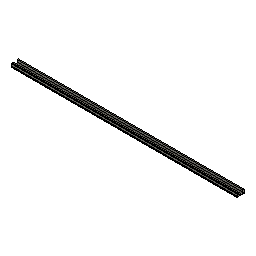
Extrusion Cover v6 200mm (Autodesk Fusion 360 design; units mm, degrees)
Autodesk Fusion 360 part; units mm, degrees
sketch "Sketch1" plane through (0, 0, 0) normal (1, 0, 0) x (0, 1, 0) in component "Cover"
sketch "Sketch2" plane through (0, 0, 0) normal (1, 0, 0) x (0, 1, 0) in component "Cover"
  line L0 (-3.5, -0.405) -> (3.5, -0.405)
  line L1 (-3.5, -0.405) -> (-3.5, -0.005)
  line L2 (3.5, -0.405) -> (3.5, -0.005)
  line L3 (-3, -0.005) -> (-3, 1.895)
  line L4 (3, -0.005) -> (3, 1.895)
  line L5 (-1.8, -0.005) -> (-1.8, 1.895)
  line L6 (1.8, -0.005) -> (1.8, 1.895)
  line L7 (-1.8, 1.895) -> (-1.8, 2.795)
  line L8 (1.8, 1.895) -> (1.8, 2.795)
  line L9 (-1.8, 2.795) -> (-3.2, 2.795)
  line L10 (1.8, 2.795) -> (3.2, 2.795)
  line L11 (-3, 1.895) -> (-3.2, 1.895)
  line L12 (3, 1.895) -> (3.2, 1.895)
  line L13 (-3.2, 2.795) -> (-3.2, 1.895)
  line L14 (3.2, 2.795) -> (3.2, 1.895)
  line L15 (-3.5, -0.005) -> (-3, -0.005)
  line L16 (-1.8, -0.005) -> (1.8, -0.005)
  line L17 (3, -0.005) -> (3.5, -0.005)
  dimension "d6" = 7
  dimension "d10" = 0.4
  dimension "d12" = 0.4
  dimension "d13" = 3
  dimension "d14" = 3
  dimension "d17" = 1.9
  dimension "d18" = 1.9
  dimension "d20" = 1.2
  dimension "d21" = 1.2
  dimension "d25" = 1.4
  dimension "d26" = 0.2
  dimension "d39" = 2.8
  dimension "d40" = 0.005
  dimension "d41" = 3.5
  constraint horizontal L0
  constraint perpendicular L0 L1
  constraint perpendicular L0 L2
  constraint perpendicular L3 L15
  constraint coincident L4.start L15
  constraint perpendicular L4 L15
  constraint coincident L5.start L15
  constraint perpendicular L5 L15
  constraint coincident L6.start L15
  constraint perpendicular L6 L15
  constraint equal L3 L5
  constraint equal L4 L6
  constraint parallel L5 L7
  constraint parallel L6 L8
  constraint equal L7 L8
  constraint perpendicular L7 L9
  constraint perpendicular L8 L10
  constraint equal L9 L10
  constraint perpendicular L3 L11
  constraint perpendicular L4 L12
  constraint equal L11 L12
  constraint collinear L15 L16
  constraint collinear L16 L17
  measures "d6" distance of L0.start L0.end
  measures "d10" distance of L0.start L1.end
  measures "d12" distance of L0.end L2.end
  measures "d13" distance of origin L3
  measures "d14" distance of origin L4
  measures "d17" vertical distance of L1.end L3.end
  measures "d18" vertical distance of L2.end L4.end
  measures "d20" distance of L3 L5
  measures "d21" distance of L4 L6
  measures "d25" distance of L7.end L9.end
  measures "d26" distance of L3.end L11.end
  measures "d39" distance of L9 L16
  measures "d40" distance of origin L16
  measures "d41" horizontal distance of origin L0.start
extrude "Extrude1" add sketch "Sketch2" against normal blind 200 in component "Cover"
fillet "Fillet1" radius 1 1 edges at (-100, 1.8, -0.005) in component "Cover"
fillet "Fillet2" radius 1 1 edges at (-100, -1.8, -0.005) in component "Cover"
chamfer "Chamfer1" distance 0.2 angle 45 1 edges at (-100, 3.2, 1.895) in component "Cover"
chamfer "Chamfer2" distance 0.2 angle 45 1 edges at (-100, -3.2, 1.895) in component "Cover"
fillet "Fillet3" radius 0.2 1 edges at (-100, -3, -0.005) in component "Cover"
fillet "Fillet4" radius 0.2 1 edges at (-100, 3, -0.005) in component "Cover"
chamfer "Chamfer3" distance 0.3 angle 45 2 edges at (-100, -3.2, 2.795) (-100, 3.2, 2.795) in component "Cover"
component "Cover" placed x (1, 0, 0) y (0, 1, 0) z (0, 0, 1) at (0, 0, 0)
equation "width_bottom = 7 mm"
equation "Bottom_radius = 0.2 mm"
equation "radius_inside = 1 mm"
equation "chamfer_inside = 0.2 mm"
equation "length = 200 mm"
equation "d6 = width_bottom"
equation "layer_height = 0.2 mm"
equation "d10 = num_layer_bottom * layer_height"
equation "num_layer_bottom = 2"
equation "d12 = num_layer_bottom * layer_height"
equation "height_below_chamfer = 1.9 mm"
equation "chamfe_angle = 60 deg"
equation "d17 = height_below_chamfer"
equation "d18 = height_below_chamfer"
equation "wall_width = 1.2 mm"
equation "d20 = wall_width"
equation "d21 = wall_width"
equation "overhang = 0.2 mm"
equation "height_overall = 2.8 mm"
equation "d25 = wall_width + overhang"
equation "d26 = overhang"
equation "d27 = -length"
equation "d30 = radius_inside"
equation "d32 = radius_inside"
equation "d33 = chamfer_inside"
equation "d34 = chamfer_inside"
equation "d36 = Bottom_radius"
equation "d38 = Bottom_radius"
equation "d39 = height_overall"
equation "d41 = width_bottom / 2"
